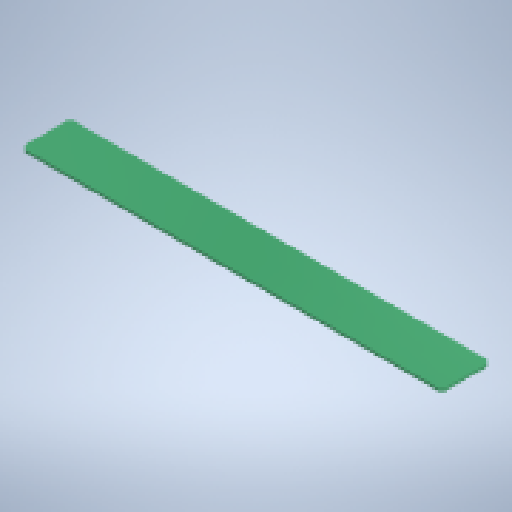
# Autodesk Inventor part: PCB
Saved by Autodesk Inventor 2023.1 (Build 271208000, 208)
## iProperties
Created: 2023-11-19
Part Number: PCB
Material: GFRC
Document SubType Name: Modeling
Designer: Vinicius
Density: 1.7 g/cm^3
Appearance: Smooth - Dark Sea Green
Author: Vinicius
Autodesk Inventor part; units mm, degrees
ref_plane "YZ Plane" through (0, 0, 0) normal (1, 0, 0) x (0, 1, 0)
ref_plane "XZ Plane" through (0, 0, 0) normal (0, 1, 0) x (-1, 0, 0)
ref_plane "XY Plane" through (0, 0, 0) normal (0, 0, 1) x (1, 0, 0)
sketch "Sketch1" plane through (0, 0, 0) normal (0, 1, 0) x (-1, 0, 0)
  line L0 (57, 7) -> (-57, 7)
  line L1 (-60, 4) -> (-60, -4)
  line L2 (-57, -7) -> (57, -7)
  line L3 (60, -4) -> (60, 4)
  line L4 (60, 7) -> (-60, -7) construction
  line L5 (-60, 7) -> (60, -7) construction
  line L6 (60, 4) -> (57, 7)
  line L7 (60, -4) -> (57, -7)
  line L8 (-60, 4) -> (-57, 7)
  line L9 (-60, -4) -> (-57, -7)
  point P0 (0, 0)
  dimension "d0" = 120
  dimension "d1" = 14
  dimension "d2" = 3
  dimension "d3" = 3
  dimension "d4" = 3
  dimension "d5" = 3
  dimension "d6" = 3
  dimension "d7" = 3
  dimension "d8" = 3
  dimension "d9" = 3
  constraints: 20 end point, 8 point on line, 2 midpoint, 2 parallel, 1 horizontal, 1 perpendicular
  measures "d0" distance of L5.end L4.end
  measures "d1" distance of L4.end L5.start
  measures "d2" distance of L3.end L4.start
  measures "d3" distance of L0.start L4.start
  measures "d4" distance of L3.start L5.end
  measures "d5" distance of L2.end L5.end
  measures "d6" distance of L1.start L5.start
  measures "d7" distance of L0.end L5.start
  measures "d8" distance of L1.end L4.end
  measures "d9" distance of L2.start L4.end
extrude "Extrusion1" add sketch "Sketch1" along normal blind 0.8
equation "\"d3\" = d2"
equation "\"d4\" = d2"
equation "\"d5\" = d4"
equation "\"d6\" = d2"
equation "\"d7\" = d6"
equation "\"d8\" = d2"
equation "\"d9\" = d8"
body "Solid1"
